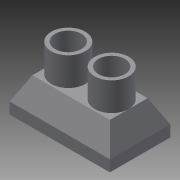
# Autodesk Inventor part: Fantest
Saved by Autodesk Inventor 2015 SP1 (Build 190203100, 203)
## iProperties
Created: 2014-12-19
Part Number: Fantest
Material: Generic
Document SubType Name: Modeling
Designer: Jack
Density: 1 g/cm^3
Appearance: Default
Author: Jack
Autodesk Inventor part; units mm, degrees
ref_plane "YZ Plane" through (0, 0, 0) normal (1, 0, 0) x (0, 1, 0)
ref_plane "XZ Plane" through (0, 0, 0) normal (0, 1, 0) x (-1, 0, 0)
ref_plane "XY Plane" through (0, 0, 0) normal (0, 0, 1) x (1, 0, 0)
sketch "Sketch1" plane through (0, 0, 0) normal (0, 0, 1) x (1, 0, 0)
  line L0 (0, 0) -> (26.5, 0)
  line L1 (26.5, 0) -> (26.5, 16)
  line L2 (26.5, 16) -> (0, 16)
  line L3 (0, 16) -> (0, 0)
  dimension "d0" = 26.5
  dimension "d1" = 16
  constraints: 8 end point, 2 horizontal, 2 perpendicular
  measures "d0" distance of L0.start L0.end
  measures "d1" distance of L0.end L1.end
extrude "Extrusion1" add sketch "Sketch1" along normal blind 3
ref_plane "Work Plane1" through (0, 0, 9) normal (0, 0, 1) x (1, 0, 0)
sketch "Sketch2" plane through (0, 0, 9) normal (0, 0, 1) x (1, 0, 0)
  line L0 (3, 13) -> (23.5, 13)
  line L1 (23.5, 13) -> (23.5, 3)
  line L2 (23.5, 3) -> (3, 3)
  line L3 (3, 3) -> (3, 13)
  line L4 (26.5, 16) -> (0, 16) projected
  line L5 (26.5, 0) -> (26.5, 16) projected
  line L6 (0, 0) -> (26.5, 0) projected
  line L7 (0, 16) -> (0, 0) projected
  dimension "d9" = 3
  dimension "d10" = 3
  dimension "d11" = 3
  dimension "d12" = 3
  constraints: 8 end point, 2 parallel, 1 horizontal, 1 perpendicular
  measures "d9" distance between parallel lines of L4 L0
  measures "d10" distance between parallel lines of L5 L1
  measures "d11" distance between parallel lines of L6 L2
  measures "d12" distance between parallel lines of L7 L3
loft "Loft1" add profiles "Sketch2" section 2 edges at (13.25, 0, 3) (26.5, 8, 3) (13.25, 16, 3) (0, 8, 3) contours L0 L1 L2 L3
sketch "Sketch3" plane through (3, 13, 9) normal (0, 0, 1) x (1, 0, 0)
  line L0 (0, 0) -> (20.5, 0) projected
  line L1 (0, -10) -> (0, 0) projected
  line L2 (20.5, 0) -> (20.5, -10) projected
  circle A0 centre (4.5, -5) radius 4.5
  circle A1 centre (16, -5) radius 4.5
  point P0 (-3, -13)
  dimension "d18" = 9
  dimension "d19" = 9
  dimension "d20" = 4.5
  dimension "d21" = 4.5
  dimension "d22" = 5
  constraints: 2 centre point, 1 horizontal alignment
  measures "d18" diameter of A0
  measures "d19" diameter of A1
  measures "d20" distance from line of L1 A0.centre
  measures "d21" distance from line of L2 A1.centre
  measures "d22" distance from line of L0 A0.centre
extrude "Extrusion2" add sketch "Sketch3" along normal blind 7.5
sketch "Sketch4" plane through (7.5, 8, 16.5) normal (0, 0, 1) x (1, 0, 0)
  circle A0 centre (0, 0) radius 4.5 projected
  circle A1 centre (11.5, 0) radius 4.5 projected
  circle A2 centre (0, 0) radius 3.5
  circle A3 centre (11.5, 0) radius 3.5
  point P0 (-7.5, -8)
  dimension "d25" = 7
  dimension "d26" = 7
  constraints: 2 centre point, 2 coincident
  measures "d25" diameter of A2
  measures "d26" diameter of A3
extrude "Extrusion3" cut sketch "Sketch4" against normal up to surface (16.5 mm away) contours A2 | A3
ref_plane "Work Plane2" through (3, 13, 7) normal (0, 0, 1) x (1, 0, 0)
sketch "Sketch5" plane through (3, 13, 7) normal (0, 0, 1) x (1, 0, 0)
  line L0 (0, -10) -> (20.5, -10)
  line L1 (20.5, -10) -> (20.5, 0)
  line L2 (20.5, 0) -> (0, 0)
  line L3 (0, 0) -> (0, -10)
  line L4 (23.5, 3) -> (-3, 3) projected
  line L5 (-3, 3) -> (-3, -13) projected
  line L6 (23.5, -13) -> (23.5, 3) projected
  line L7 (-3, -13) -> (23.5, -13) projected
  dimension "d30" = 3
  dimension "d31" = 3
  dimension "d32" = 3
  dimension "d33" = 3
  constraints: 8 end point, 2 parallel, 1 horizontal, 1 perpendicular
  measures "d30" distance between parallel lines of L4 L2
  measures "d31" distance between parallel lines of L5 L3
  measures "d32" distance between parallel lines of L6 L1
  measures "d33" distance between parallel lines of L7 L0
sketch "Sketch6" plane through (0, 0, 0) normal (0, 0, -1) x (-1, 0, 0)
  line L0 (0, 0) -> (-26.5, 0) projected
  line L1 (0, 16) -> (0, 0) projected
  line L2 (-26.5, 16) -> (0, 16) projected
  line L3 (-26.5, 0) -> (-26.5, 16) projected
  line L4 (-2, 14) -> (-24.5, 14)
  line L5 (-24.5, 14) -> (-24.5, 2)
  line L6 (-24.5, 2) -> (-2, 2)
  line L7 (-2, 2) -> (-2, 14)
  dimension "d34" = 2
  dimension "d35" = 2
  dimension "d36" = 2
  dimension "d37" = 2
  constraints: 8 end point, 2 parallel, 1 horizontal, 1 perpendicular
  measures "d34" distance between parallel lines of L0 L6
  measures "d35" distance between parallel lines of L3 L5
  measures "d36" distance between parallel lines of L2 L4
  measures "d37" distance between parallel lines of L1 L7
loft "Loft2" cut profiles "Sketch6", "Sketch5" contours L7 L6 L5 L4 / L3 L2 L1 L0
body "Solid1"
